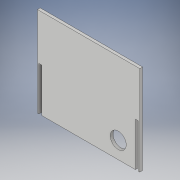
# Autodesk Inventor part: back
Saved by Autodesk Inventor 2018 (Build 220112000, 112)
## iProperties
Created: 2018-04-09
Part Number: back
Material: Generic
Document SubType Name: Modeling
Designer: guita
Density: 1 g/cm^3
Appearance: Default
Author: guita
Autodesk Inventor part; units mm, degrees
ref_plane "YZ Plane" through (0, 0, 0) normal (1, 0, 0) x (0, 1, 0)
ref_plane "XZ Plane" through (0, 0, 0) normal (0, 1, 0) x (-1, 0, 0)
ref_plane "XY Plane" through (0, 0, 0) normal (0, 0, 1) x (1, 0, 0)
sketch "Sketch1" plane through (0, 0, 0) normal (0, 0, 1) x (1, 0, 0)
  line L0 (-203.2, 0) -> (-203.2, 177.8)
  line L1 (-203.2, 177.8) -> (0, 177.8)
  line L2 (0, 177.8) -> (0, 0)
  line L3 (-203.2, 0) -> (-200.025, 0)
  line L4 (-200.025, 0) -> (-200.025, 86.614)
  line L5 (0, 0) -> (-3.175, 0)
  line L6 (-3.175, 0) -> (-3.175, 86.614)
  line L7 (-9.525, 86.614) -> (-3.175, 86.614)
  line L8 (-193.675, 86.614) -> (-200.025, 86.614)
  line L9 (-200.025, 0) -> (-203.2, 0)
  line L10 (0, 0) -> (-3.175, 0)
  line L11 (-9.525, 0) -> (-193.675, 0)
  circle A0 centre (-42.8625, 33.3375) radius 15.875
  line L12 (-9.525, 43.307) -> (-8.7313, 43.307)
  line L13 (-8.7313, 43.307) -> (-8.7313, 86.614)
  line L14 (-8.7313, 43.307) -> (-8.7313, 0)
  line L15 (-8.7313, 0) -> (-9.525, 0)
  line L16 (-194.4688, 43.307) -> (-194.4688, 86.614)
  line L17 (-194.4688, 43.307) -> (-194.4688, 0)
  line L18 (-194.4688, 0) -> (-193.675, 0)
  dimension "d0" = 203.2
  dimension "d7" = 31.75
  constraints: 38 end point, 10 perpendicular, 4 horizontal, 4 parallel, 4 point on line, 1 centre point
  measures "d0" distance of L0.end L1.end
  measures "d7" diameter of A0
extrude "Extrusion1" add sketch "Sketch1" along normal blind 5.5563
body "Solid1"
